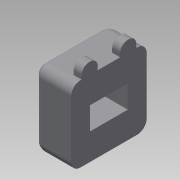
# Autodesk Inventor part: pig_face
Saved by Autodesk Inventor 2015 (Build 190159000, 159)
## iProperties
Created: 2016-04-29
Part Number: pig_face
Material: Generic
Document SubType Name: Modeling
Designer: Luke Good
Density: 1 g/cm^3
Appearance: Default
Author: Luke Good
Autodesk Inventor part; units mm, degrees
ref_plane "YZ Plane" through (0, 0, 0) normal (1, 0, 0) x (0, 1, 0)
ref_plane "XZ Plane" through (0, 0, 0) normal (0, 1, 0) x (-1, 0, 0)
ref_plane "XY Plane" through (0, 0, 0) normal (0, 0, 1) x (1, 0, 0)
sketch "Sketch1" plane through (0, 0, 0) normal (0, 0, 1) x (1, 0, 0)
  line L0 (6.35, -12.6955) -> (-3.175, -12.6955)
  line L1 (-6.35, -9.5205) -> (-6.35, 9.5205)
  line L2 (-3.175, 12.6955) -> (6.35, 12.6955)
  line L3 (6.35, 12.6955) -> (6.35, -12.6955)
  line L4 (6.35, -12.6955) -> (-6.35, 12.6955) construction
  line L5 (-6.35, -12.6955) -> (6.35, 12.6955) construction
  arc A0 (-3.175, 12.6955) -> (-6.35, 9.5205) centre (-3.175, 9.5205) ccw
  arc A1 (-6.35, -9.5205) -> (-3.175, -12.6955) centre (-3.175, -9.5205) ccw
  point P0 (0, 0)
  dimension "d0" = 12.7
  dimension "d1" = 3.175
  constraints: 12 end point, 4 point on circle, 4 point on line, 4 tangent, 2 centre point, 2 midpoint, 2 parallel, 1 equal radius, 1 horizontal, 1 perpendicular
  measures "d0" distance of L4.end L2.end
  measures "d1" radius of A0
extrude "Extrusion1" add sketch "Sketch1" along normal blind 25.4
fillet "Fillet1" radius 3.175 10 edges at (-6.35, 0, 25.4) (-5.4201, -11.7656, 25.4) (1.5875, -12.6955, 25.4) (1.5875, 12.6955, 25.4) (-5.4201, 11.7656, 25.4) (-5.4201, 11.7656, 0) (1.5875, 12.6955, 0) (-5.4201, -11.7656, 0) (1.5875, -12.6955, 0) (-6.35, 0, 0)
sketch "Sketch2" plane through (-3.175, 12.6955, 3.175) normal (0, 1, 0) x (1, 0, 0)
  circle A0 centre (2.6716, -16.206) radius 2.54
  line L0 (0, 0) -> (0, -19.05) projected
  line L1 (9.525, 0) -> (9.525, -19.05) projected
  circle A1 centre (2.6716, -2.844) radius 2.54
  point P0 (3.175, 3.175)
  dimension "d5" = 5.08
  constraints: 2 centre point
  measures "d5" diameter of A0
extrude "Extrusion2" add sketch "Sketch2" along normal blind 12.7
sketch "Sketch3" plane through (-6.35, -9.5205, 3.175) normal (-1, 0, 0) x (0, 0, 1)
  line L0 (4.445, 6.9805) -> (14.605, 12.0605) construction
  line L1 (14.605, 6.9805) -> (4.445, 12.0605) construction
  line L2 (3.175, 5.7105) -> (3.175, 13.3305)
  line L3 (15.875, 13.3305) -> (15.875, 5.7105)
  line L4 (15.875, 5.0755) -> (3.175, 13.9655) construction
  line L5 (3.175, 5.0755) -> (15.875, 13.9655) construction
  line L6 (3.175, 13.3305) -> (15.875, 13.3305)
  line L7 (15.875, 13.3305) -> (15.875, 5.7105)
  line L8 (15.875, 5.7105) -> (3.175, 5.7105)
  line L9 (3.175, 5.7105) -> (3.175, 13.3305)
  line L10 (3.175, 13.3305) -> (15.875, 5.7105) construction
  line L11 (15.875, 13.3305) -> (3.175, 5.7105) construction
  point P0 (-3.175, 9.5205)
  point P1 (9.525, 9.5205)
  point P2 (15.875, 12.0605)
  point P3 (15.875, 6.9805)
  dimension "d25" = 7.62
  constraints: 24 end point, 6 midpoint, 3 parallel, 1 horizontal, 1 perpendicular
  measures "d25" distance of L3.start L3.end
extrude "Extrusion3" cut sketch "Sketch3" against normal blind 12.7
sketch "Sketch4" plane through (-0.5034, 25.3955, 19.381) normal (0, 1, 0) x (1, 0, 0)
  line L0 (-9.3616, 22.1264) -> (11.0198, 22.1264)
  line L1 (11.0198, 22.1264) -> (11.0198, -9.2368)
  line L2 (11.0198, -9.2368) -> (-9.3616, -9.2368)
  line L3 (-9.3616, -9.2368) -> (-9.3616, 22.1264)
  point P0 (0.5034, 19.381)
  constraints: 8 end point, 2 parallel, 1 horizontal, 1 perpendicular
extrude "Extrusion4" cut sketch "Sketch4" against normal blind 12.7
sketch "Sketch5" plane through (-3.175, 12.6955, 3.175) normal (0, 1, 0) x (1, 0, 0)
  line L0 (6.852, -0.3615) -> (9.5509, -0.3615)
  line L1 (9.5509, -0.3615) -> (9.5509, -5.7593)
  line L2 (9.5509, -5.7593) -> (6.852, -5.7593)
  line L3 (6.852, -5.7593) -> (6.852, -0.3615)
  line L4 (6.852, -0.3615) -> (9.5509, -5.7593) construction
  line L5 (9.5509, -0.3615) -> (6.852, -5.7593) construction
  line L6 (0, 0) -> (0, -19.05) projected
  line L7 (9.525, 0) -> (9.525, -19.05) projected
  line L8 (6.852, -18.6885) -> (9.5509, -18.6885)
  line L9 (9.5509, -18.6885) -> (9.5509, -13.2907)
  line L10 (9.5509, -13.2907) -> (6.852, -13.2907)
  line L11 (6.852, -13.2907) -> (6.852, -18.6885)
  line L12 (6.852, -18.6885) -> (9.5509, -13.2907) construction
  line L13 (9.5509, -18.6885) -> (6.852, -13.2907) construction
  point P0 (3.175, 3.175)
  point P1 (8.2015, -3.0604)
  point P2 (8.2015, -15.9896)
  constraints: 24 end point, 4 midpoint, 2 parallel, 1 horizontal, 1 perpendicular
extrude "Extrusion5" add sketch "Sketch5" along normal blind 3.81
fillet "Fillet2" radius 2.54 4 edges at (5.0265, 16.5055, 8.9343) (5.0265, 16.5055, 3.5365) (5.0265, 16.5055, 16.4657) (5.0265, 16.5055, 21.8635)
sketch "Sketch7" plane through (-6.35, -9.5205, 3.175) normal (-1, 0, 0) x (0, 0, 1)
  circle A0 centre (3.0142, 16.7412) radius 1.27
  circle A1 centre (15.8269, 16.7412) radius 1.27
  point P0 (-3.175, 9.5205)
  dimension "d26" = 2.54
  dimension "d27" = 2.54
  constraints: 2 centre point
  measures "d26" diameter of A0
  measures "d27" diameter of A1
extrude "Extrusion7" cut sketch "Sketch7" against normal blind 1.27
body "Solid1"
